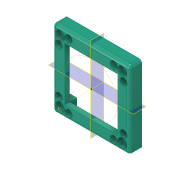
# Autodesk Inventor part: 10_Lid_1x1_v3
Saved by Autodesk Inventor 2022 (Build 260153000, 153)
## iProperties
Created: 2019-07-01
Part Number: 10_Lid_1x1_v3
Material: Generic
Document SubType Name: Modeling
Designer: diederichbenedict
Density: 1 g/cm^3
Appearance: IPHT_Türkis
Author: diederichbenedict
Autodesk Inventor part; units mm, degrees
ref_plane "YZ Plane" through (0, 0, 0) normal (1, 0, 0) x (0, 1, 0)
ref_plane "XZ Plane" through (0, 0, 0) normal (0, 1, 0) x (-1, 0, 0)
ref_plane "Work Plane1" through (0, 41.8, -12.9) normal (0, 0, 1) x (1, 0, 0)
sketch "Sketch1" plane through (0, 41.8, -12.9) normal (0, 0, 1) x (1, 0, 0)
  line L0 (3.85, 0.3752) -> (3.85, 4) construction
  line L1 (3.85, 4) -> (-2, 4) construction
  arc A0 (-2, 4) -> (-4, 2) centre (-2, 2) ccw construction
  line L2 (-4, 2) -> (-4, -3.85) construction
  line L3 (-4, -3.85) -> (-0.3752, -3.85) construction
  line L4 (-2, 4) -> (43.8, 4)
  line L5 (45.8, 2) -> (45.8, -43.8)
  line L6 (43.8, -45.8) -> (-2, -45.8)
  line L7 (-4, -43.8) -> (-4, 2)
  line L8 (40.3, -37.8) -> (40.3, -4)
  line L9 (37.8, -1.5) -> (4, -1.5)
  line L10 (1.5, -4) -> (1.5, -37.8)
  line L11 (4, -40.3) -> (37.8, -40.3)
  line L12 (37.8, -40.3) -> (40.3, -37.8)
  line L13 (4, -40.3) -> (1.5, -37.8)
  line L14 (4, -1.5) -> (1.5, -4)
  line L15 (40.3, -4) -> (37.8, -1.5)
  arc A1 (45.8, 2) -> (43.8, 4) centre (43.8, 2) ccw
  arc A2 (43.8, -45.8) -> (45.8, -43.8) centre (43.8, -43.8) ccw
  arc A3 (-4, -43.8) -> (-2, -45.8) centre (-2, -43.8) ccw
  arc A4 (-2, 4) -> (-4, 2) centre (-2, 2) ccw
  circle A5 centre (1, -1) radius 1.4
  circle A6 centre (40.8, -1) radius 1.4
  circle A7 centre (40.8, -40.8) radius 1.4
  circle A8 centre (1, -40.8) radius 1.4
  circle A9 centre (20.9, -20.9) radius 19.4 construction
  line L16 (3.85, -3.85) -> (3.85, -37.95)
  line L17 (3.85, -37.95) -> (37.95, -37.95)
  line L18 (37.95, -37.95) -> (37.95, -3.85)
  line L19 (37.95, -3.85) -> (3.85, -3.85)
  arc A10 (2.2654, -1.2094) -> (1.2094, -2.2654) centre (0.9, -0.9) ccw projected
  line L20 (2.2654, -1.2094) -> (3.85, 0.3752) projected
  line L21 (-0.3752, -3.85) -> (1.2094, -2.2654) projected
  point P0 (45.8, -45.8)
  point P1 (45.8, 4)
  point P2 (-4, -45.8)
  point P3 (40.3, -40.3)
  point P4 (40.3, -1.5)
  point P5 (1.5, -1.5)
  point P6 (1.5, -40.3)
  point P7 (40.8, -1)
  dimension "d55" = 2.8
  dimension "d34" = 49.8
  dimension "d35" = 49.8
  dimension "d36" = 5.5
  dimension "d37" = 2.5
  dimension "d38" = 2.5
  dimension "d39" = 2.5
  dimension "d40" = 2.5
  dimension "d41" = 2.5
  dimension "d42" = 2.5
  dimension "d43" = 2.5
  dimension "d44" = 2.5
  dimension "d45" = 2
  dimension "d46" = 5
  dimension "d47" = 5
  dimension "d48" = 5
  dimension "d49" = 5
  dimension "d51" = 5
  dimension "d52" = 0.5
  dimension "d53" = 5
  dimension "d54" = 5
  dimension "d56" = 2.8
  dimension "d57" = 2.8
  dimension "d58" = 2.8
  dimension "d90" = 7.85
  constraints: 32 end point, 14 point on line, 11 tangent, 8 centre point, 8 point on circle, 6 parallel, 3 coincident, 3 equal radius, 3 perpendicular, 1 horizontal, 8 other
  measures "d34" distance of point (45.8, -45.8) point (-4, -45.8)
  measures "d35" distance of point (45.8, 4) point (45.8, -45.8)
  measures "d36" distance between parallel lines of L5 L8
  measures "d37" distance of L11.end point (40.3, -40.3)
  measures "d38" distance of L8.start point (40.3, -40.3)
  measures "d39" distance of L11.start point (1.5, -40.3)
  measures "d40" distance of L10.end point (1.5, -40.3)
  measures "d41" distance of L9.end point (1.5, -1.5)
  measures "d42" distance of L10.start point (1.5, -1.5)
  measures "d43" distance of L8.end point (40.3, -1.5)
  measures "d44" distance of L9.start point (40.3, -1.5)
  measures "d45" radius of A1
  measures "d46" distance from line of point (1, -40.8) L7
  measures "d47" distance from line of L6 point (1, -40.8)
  measures "d48" distance from line of L5 point (40.8, -40.8)
  measures "d49" distance from line of L6 point (40.8, -40.8)
  measures "d51" distance from line of L4 point (40.8, -1)
  measures "d52" distance from line of point (1, -1) L10
  measures "d53" distance from line of L2 point (1, -1)
  measures "d54" distance from line of L1 point (1, -1)
  measures "d56" diameter of A6
  measures "d57" diameter of A7
  measures "d58" diameter of A8
  measures "d90" distance between parallel lines of L7 L16
extrude "Extrusion1" add sketch "Sketch1" along normal blind 7.7 contours L4 A1 L5 A2 L6 A3 L7 A4 | L12 L11 L13 L10 L14 L9 L15 L8 | A5 A10
fillet "Fillet1" radius 2 8 edges at (20.9, -4, -5.2) (45.2142, -3.4142, -5.2) (45.8, 20.9, -5.2) (45.2142, 45.2142, -5.2) (20.9, 45.8, -5.2) (-3.4142, 45.2142, -5.2) (-4, 20.9, -5.2) (-3.4142, -3.4142, -5.2)
sketch "Sketch3" plane through (0, 41.8, -5.2) normal (0, 0, 1) x (1, 0, 0)
  circle A0 centre (20.9, -20.9) radius 16.9 construction
  point P0 (0, -41.8)
  constraints: 1 centre point
sketch "Sketch4" plane through (0, 41.8, -5.2) normal (0, 0, 1) x (1, 0, 0)
  line L0 (37.95, -37.95) -> (37.95, -3.85) projected
  line L1 (37.95, -3.85) -> (3.85, -3.85) projected
  line L2 (3.85, -3.85) -> (3.85, -37.95) projected
  line L3 (3.85, -37.95) -> (37.95, -37.95) projected
  circle A0 centre (40.9, -0.9) radius 2.75 projected
  circle A1 centre (0.9, -40.9) radius 2.75 projected
  circle A2 centre (0.9, -0.9) radius 2.75 projected
  circle A3 centre (40.9, -40.9) radius 2.75 projected
  line L4 (34.3452, 2) -> (7.4548, 2) projected
  line L5 (43.8, -34.3452) -> (43.8, -7.4548) projected
  line L6 (7.4548, -43.8) -> (34.3452, -43.8) projected
  line L7 (-2, -7.4548) -> (-2, -34.3452) projected
  arc A4 (34.3452, 2) -> (36.4548, 2) centre (35.4, -0.1) ccw projected
  line L8 (43.8, 2) -> (36.4548, 2) projected
  line L9 (43.8, -5.3452) -> (43.8, 2) projected
  arc A5 (43.8, -5.3452) -> (43.8, -7.4548) centre (41.7, -6.4) ccw projected
  arc A6 (43.8, -34.3452) -> (43.8, -36.4548) centre (41.7, -35.4) ccw projected
  line L10 (43.8, -43.8) -> (43.8, -36.4548) projected
  line L11 (36.4548, -43.8) -> (43.8, -43.8) projected
  arc A7 (36.4548, -43.8) -> (34.3452, -43.8) centre (35.4, -41.7) ccw projected
  arc A8 (7.4548, -43.8) -> (5.3452, -43.8) centre (6.4, -41.7) ccw projected
  line L12 (-2, -43.8) -> (5.3452, -43.8) projected
  line L13 (-2, -36.4548) -> (-2, -43.8) projected
  arc A9 (-2, -36.4548) -> (-2, -34.3452) centre (0.1, -35.4) ccw projected
  arc A10 (-2, -7.4548) -> (-2, -5.3452) centre (0.1, -6.4) ccw projected
  line L14 (-2, 2) -> (-2, -5.3452) projected
  line L15 (5.3452, 2) -> (-2, 2) projected
  arc A11 (5.3452, 2) -> (7.4548, 2) centre (6.4, -0.1) ccw projected
hole "Hole2" at (40.9, 40.9, -5.2) at (40.9, 0.9, -5.2) at (0.9, 0.9, -5.2) at (0.9, 40.9, -5.2) direction (0, 0, -1) diameter 3.2 depth 12 tip angle 118 counterbore diameter 6 counterbore depth 3.1
chamfer "Chamfer2" distance 4.6 angle 45 2 edges at (3.85, 20.9, -12.9) (37.95, 20.9, -12.9)
sketch "Sketch9" plane through (37.95, 3.85, -5.2) normal (-1, 0, 0) x (0, 0, 1)
  line L0 (-7.7, 0) -> (-3.1, 0) projected
  line L1 (-3.1, 34.1) -> (-7.7, 34.1) projected
  line L2 (-3.1, 0) -> (-7.7, -4.6)
  line L3 (-7.7, 39.95) -> (-7.7, -5.85) projected
  line L4 (-3.1, 0) -> (3.4054, 0) construction
  line L5 (-7.7, -4.6) -> (-7.7, 0)
  line L6 (-3.1, 34.1) -> (-7.7, 38.7)
  line L7 (-3.1, 34.1) -> (3.4054, 34.1) construction
  line L8 (-7.7, 38.7) -> (-7.7, 34.1)
  line L9 (-7.7, 34.1) -> (-3.1, 34.1)
  point P0 (5.2, -3.85)
  point P1 (-7.7, -5.85)
  dimension "d91" = 135
  dimension "d92" = 135
  constraints: 14 end point, 2 equal length, 2 horizontal, 2 vertical, 1 collinear, 3 other
  measures "d91" angle of L2 L4
  measures "d92" angle of L7 L6
extrude "Extrusion3" cut sketch "Sketch9" along normal up to surface (34.1 mm away)
sketch "Sketch14" plane through (0, 41.8, -5.2) normal (0, 0, 1) x (1, 0, 0)
  arc A0 (1.6681, -43.8) -> (-2, -40.1319) centre (0.9, -40.9) ccw construction
  line L0 (40.1319, -43.8) -> (1.6681, -43.8) construction
  arc A1 (43.8, -40.1319) -> (40.1319, -43.8) centre (40.9, -40.9) ccw construction
  line L1 (43.8, -1.6681) -> (43.8, -40.1319) construction
  arc A2 (40.1319, 2) -> (43.8, -1.6681) centre (40.9, -0.9) ccw construction
  line L2 (1.6681, 2) -> (40.1319, 2) construction
  arc A3 (-2, -1.6681) -> (1.6681, 2) centre (0.9, -0.9) ccw construction
  line L3 (-2, -40.1319) -> (-2, -1.6681) construction
  line L4 (3.85, -3.85) -> (37.95, -3.85) construction
  line L5 (37.95, -3.85) -> (37.95, -37.95) construction
  line L6 (37.95, -37.95) -> (3.85, -37.95) construction
  line L7 (3.85, -37.95) -> (3.85, -3.85) construction
  point P0 (0, -41.8)
  point P1 (6.4, -0.1)
  point P2 (0.1, -6.4)
  point P3 (0.1, -35.4)
  point P4 (6.4, -41.7)
  point P5 (35.4, -41.7)
  point P6 (41.7, -35.4)
  point P7 (41.7, -6.4)
  point P8 (35.4, -0.1)
hole "Hole6" at (6.4, 41.7, -5.2) at (0.1, 35.4, -5.2) at (0.1, 6.4, -5.2) at (6.4, 0.1, -5.2) at (35.4, 0.1, -5.2) at (41.7, 6.4, -5.2) at (41.7, 35.4, -5.2) at (35.4, 41.7, -5.2) direction (0, 0, -1) diameter 4.7 end through all
ref_plane "Work Plane5" through (20.9, -2, -12.9) normal (-1, 0, 0) x (0, 0, 1)
ref_plane "Work Plane6" through (-2, 20.9, -12.9) normal (0, -1, 0) x (1, 0, 0)
equation "\"d38\" = d37"
equation "\"d39\" = d37"
equation "\"d40\" = d39"
equation "\"d41\" = d37"
equation "\"d42\" = d41"
equation "\"d43\" = d37"
equation "\"d44\" = d43"
body "Solid1"
